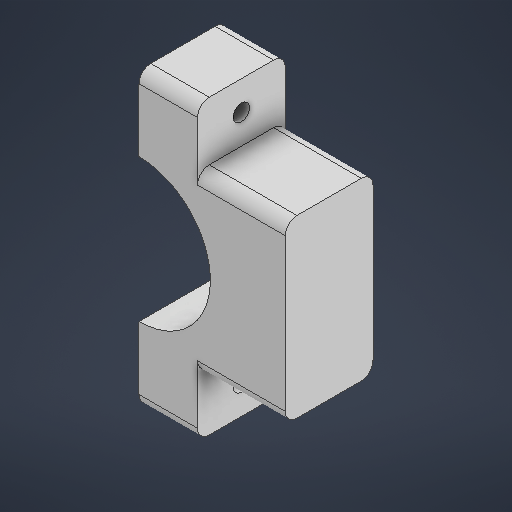
# Autodesk Inventor part: motor kapak1
Saved by Autodesk Inventor 2026.1 (Build 301233020, 233B)
## iProperties
Created: 2026-04-17
Part Number: motor kapak1
Material: Generic
Document SubType Name: Modeling
Designer: kadir
Density: 1 g/cm^3
Appearance: Default
Author: kadir
Autodesk Inventor part; units mm, degrees
ref_plane "YZ Plane" through (0, 0, 0) normal (1, 0, 0) x (0, 1, 0)
ref_plane "XZ Plane" through (0, 0, 0) normal (0, 1, 0) x (-1, 0, 0)
ref_plane "XY Plane" through (0, 0, 0) normal (0, 0, 1) x (1, 0, 0)
sketch "Sketch1" plane through (0, 0, 0) normal (0, 0, 1) x (1, 0, 0)
  line L0 (0, 0) -> (25, 0)
  line L1 (25, 0) -> (25, 30)
  line L2 (25, 30) -> (0, 30)
  line L3 (0, 30) -> (0, 0)
  circle A0 centre (0, 15) radius 12.2
  point P0 (0, 27.2)
  point P1 (0, 2.8)
  dimension "d0" = 25
  dimension "d1" = 30
  dimension "d2" = 24.4
  constraints: 8 end point, 2 parallel, 1 centre point, 1 horizontal, 1 midpoint, 1 perpendicular
  measures "d0" distance of L2.end L1.end
  measures "d1" distance of L1.end L0.end
  measures "d2" diameter of A0
extrude "Extrusion1" add sketch "Sketch1" along normal blind 15 contours L3 A0 L2 L1 L0
sketch "Sketch2" plane through (0, 30, 0) normal (0, 1, 0) x (1, 0, 0)
  line L0 (0, 0) -> (10, 0)
  line L1 (10, 0) -> (10, -15)
  line L2 (10, -15) -> (0, -15)
  line L3 (0, -15) -> (0, 0)
  dimension "d5" = 10
  dimension "d6" = 15
  constraints: 8 end point, 2 parallel, 1 horizontal, 1 perpendicular
  measures "d5" distance of L1.end L2.end
  measures "d6" distance of L0.end L1.end
extrude "Extrusion2" add sketch "Sketch2" along normal blind 10
sketch "Sketch3" plane through (0, 0, 0) normal (0, -1, 0) x (1, 0, 0)
  line L0 (25, 15) -> (10, 15) projected
  line L1 (0, 0) -> (10, 0)
  line L2 (10, 0) -> (10, 15)
  line L3 (10, 15) -> (0, 15)
  line L4 (0, 15) -> (0, 0)
  constraints: 8 end point, 2 parallel, 1 horizontal, 1 perpendicular
extrude "Extrusion3" add sketch "Sketch3" along normal blind 10
sketch "Sketch4" plane through (0, 27.2, 0) normal (-1, 0, 0) x (0, 0, 1)
  circle A0 centre (7.5, 7.8) radius 1.4
  line L0 (0, 12.8) -> (0, 0) projected
  line L1 (0, 12.8) -> (15, 12.8) projected
  line L2 (0, 0) -> (0, -24.4) projected
  line L3 (0, -12.2) -> (15, -12.2)
  line L4 (15, -27.2) -> (15, 2.8) projected
  circle A1 centre (7.5, -32.2) radius 1.4
  point P0 (0, -27.2)
  point P1 (7.5, 12.8)
  dimension "d11" = 2.8
  dimension "d12" = 7.5
  dimension "d13" = 5
  constraints: 3 midpoint, 2 centre point, 2 end point, 1 symmetric about line, 1 other
  measures "d11" diameter of A0
  measures "d12" distance from line of L0 A0.centre
  measures "d13" distance of point (7.5, 12.8) A0.centre
extrude "Extrusion4" cut sketch "Sketch4" against normal through all
fillet "Fillet1" radius 2 2 edges at (5, 40, 0) (5, 40, 15)
fillet "Fillet2" radius 2 1 edges at (5, -10, 0)
fillet "Fillet3" radius 2 1 edges at (5, -10, 15)
fillet "Fillet4" radius 2 4 edges at (17.5, 30, 15) (17.5, 30, 0) (17.5, 0, 15) (17.5, 0, 0)
body "Solid1"
